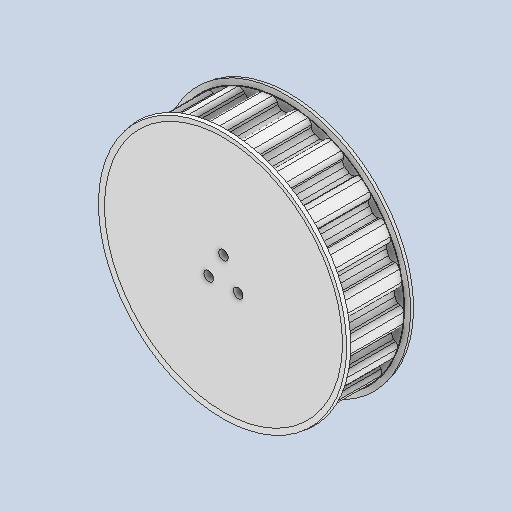
# Autodesk Inventor part: 동기식 풀리2
Saved by Autodesk Inventor 2025.3 (Build 293356030, 356C)
## iProperties
CustomPartVersion: 1
Created: 2025-09-07
Part Number: 동기식 풀리2
Material: PLA+ filament
Document SubType Name: Modeling
Designer: MSI
Density: 1.23 g/cm^3
Appearance: 일반
Mass: 146.508 g
Surface Area: 216.244 cm^2
Volume: 119.112 cm^3
Author: MSI
Autodesk Inventor part; units mm, degrees
ref_plane "YZ Plane" through (0, 0, 0) normal (1, 0, 0) x (0, 1, 0)
ref_plane "XZ Plane" through (0, 0, 0) normal (0, 1, 0) x (-1, 0, 0)
ref_plane "XY Plane" through (0, 0, 0) normal (0, 0, 1) x (1, 0, 0)
sketch "풀리 스케치" plane through (0, 0, 0) normal (0, 0, 1) x (1, 0, 0)
  circle A0 centre (0, 0) radius 42.4466 construction
  circle A1 centre (0, 0) radius 41.7608
  circle A2 centre (0, 0) radius 38.7128
  line L0 (-3.1613, 41.641) -> (-2.0955, 38.7128)
  line L1 (-2.0955, 38.7128) -> (2.0955, 38.7128)
  line L2 (2.0955, 38.7128) -> (3.1613, 41.641)
  line L3 (0, 0) -> (0, 41.7608) construction
  point P0 (0, 38.7128)
  dimension "d0" = 84.8932
  dimension "d1" = 0.6858
  dimension "d2" = 3.048
  dimension "d3" = 40
  dimension "d4" = 4.191
  constraints: 8 end point, 3 coincident, 3 point on circle, 2 centre point, 1 horizontal, 1 midpoint, 1 point on line, 1 vertical, 1 vertical alignment, 3 other
  measures "d0" diameter of A0
  measures "d1" radial gap between concentric circles of A0 A1
  measures "d3" angle of L2 L0
  measures "d4" distance of L0.end L1.end
extrude "기본 본체" add sketch "풀리 스케치" along normal mid plane 20.32 contours A2 | A1 L0 L1 L2 | L2 L1 L0 A1
extrude "톱니" cut sketch "풀리 스케치" along normal through all both and the other way through all contours L2 L1 L0 A1 picked at (0, 40.7359)
fillet "Fillet" radius 1.6002 2 edges at (2.0955, 38.7128, 0) (-2.0955, 38.7128, 0)
fillet "Fillet" radius 1.6002 4 edges at (-3.1613, 41.641, 5.08) (-3.1613, 41.641, -5.08) (3.1613, 41.641, 5.08) (3.1613, 41.641, -5.08)
pattern_circular "Teeth" count 21 over 360 about axis through (0, 0, -10) along (0, 0, 1) of "톱니", "Fillet"
pulley flange "왼쪽 플랜지" diameter 83.5216 height 2.032 thickness 1.27 bend angle 10 centre (0, 0, -10.16) toward (0, 0, -1)
pulley flange "오른쪽 플랜지" diameter 83.5216 height 2.032 thickness 1.27 bend angle 10 centre (0, 0, 10.16) toward (0, 0, 1)
sketch "스케치2" plane through (0, 0, 11.43) normal (0, 0, 1) x (1, 0, 0)
  line L0 (0, 0) -> (0, 6) construction
  dimension "d17" = 6
  constraints: 2 end point, 1 vertical
  measures "d17" distance of L0.start L0.end
hole "구멍1" at (0, 6, 11.43) direction (0, 0, -1) diameter 3.4 end through all clearance for "Flat Head Machine Screw" size "M3" standard "Ansi Metric M Profile"
pattern_circular "원형 패턴2" count 3 over 360 about axis through (0, 0, -10) along (0, 0, 1) of "구멍1"
equation "\"d1\" = da_a"
equation "\"d2\" = da_hg"
equation "\"d3\" = 2 * da_fi"
equation "\"d4\" = da_bw"
equation "\"d5\" = da_bf"
equation "\"d7\" = da_bf"
equation "\"d9\" = da_rb"
equation "\"d10\" = da_rt"
equation "\"da_pb\" = 12.7"
equation "\"da_fi\" = 20deg"
equation "\"da_hg\" = 3.048"
equation "\"da_bw\" = 4.191"
equation "\"da_rb\" = 1.6002"
equation "\"da_rt\" = 1.6002"
equation "\"da_a\" = 0.6858"
equation "\"da_bf\" = 20.32"
equation "\"da_wf\" = 1.27"
equation "\"da_hf\" = 2.032"
body "Solid1"
